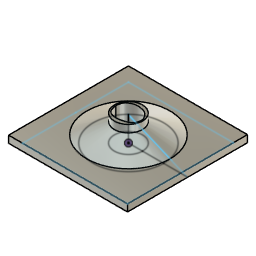
base secador v4 (Autodesk Fusion 360 design; units mm, degrees)
Autodesk Fusion 360 part; units mm, degrees
note: some values were not read from the file. Set by a fixed rule: which face or edge a step refers to.
sketch "Esboço1" plane through (0, 0, 0) normal (0, 0, 1) x (1, 0, 0)
  circle A0 centre (0, 0) radius 20
  dimension "d1" = 40
  constraint coincident A0.centre origin
  measures "d1" diameter of A0
sketch "Esboço2" plane through (0, 0, 0) normal (0, 0, 1) x (1, 0, 0)
  circle A0 centre (0, 0) radius 50
  dimension "d2" = 100
  constraint coincident A0.centre origin
  measures "d2" diameter of A0
sketch "Esboço3" plane through (0, 0, 0) normal (0, 1, 0) x (1, 0, 0)
  line L0 (0, 0) -> (82.8268, 0)
  line L1 (0, 0) -> (0, -35)
  line L2 (0, -35) -> (82.8268, 0)
  dimension "d3" = 35
  constraint coincident L0.start L1.start
  constraint horizontal L0
  constraint perpendicular L0 L1
  measures "d3" distance of L0.start L1.end
sketch "Esboço4" plane through (0, 0, 0) normal (0, 0, 1) x (1, 0, 0)
  line L0 (-75, 0) -> (-75, -75.6512)
  line L1 (-75, -75.6512) -> (74.376, -75.6512)
  line L2 (74.376, -75.6512) -> (74.376, 75.0489)
  line L3 (74.376, 75.0489) -> (-75, 75.0489)
  line L4 (-75, 75.0489) -> (-75, 0)
  constraint vertical L0
  constraint perpendicular L0 L1
  constraint perpendicular L1 L2
  constraint perpendicular L2 L3
  constraint perpendicular L1 L4
sketch "Esboço5" plane through (0, 0, 0) normal (0, 0, 1) x (1, 0, 0)
sketch "Esboço6" plane through (0, 0, 0) normal (0, 0, 1) x (1, 0, 0)
  spline S0 degree 5 poles (-18, 0) (-17.9953, 0.0513) (-17.984, 0.1676) (-17.9623, 0.4003) (-17.9267, 0.8654) (-17.8678, 1.7) (-17.7839, 2.7196) (-17.6589, 3.8334) (-17.4725, 4.9731) (-17.2029, 6.0968) (-16.8288, 7.1809) (-16.3314, 8.2159) (-15.6972, 9.2009) (-14.9196, 10.1381) (-14.0019, 11.0281) (-12.9584, 11.8645) (-11.8115, 12.6372) (-10.5887, 13.3334) (-9.3199, 13.9401) (-8.034, 14.4456) (-6.7566, 14.8417) (-5.5066, 15.1253) (-4.2932, 15.3009) (-3.115, 15.3808) (-1.9633, 15.3811) (-0.8249, 15.3201) (0.3149, 15.2144) (1.47, 15.0767) (2.6502, 14.9128) (3.8584, 14.7182) (5.0898, 14.479) (6.3344, 14.1757) (7.5785, 13.787) (8.8057, 13.293) (9.9993, 12.6789) (11.1437, 11.9389) (12.2256, 11.079) (13.236, 10.121) (14.1689, 9.0959) (15.0205, 8.0399) (15.7884, 6.9891) (16.4705, 5.9746) (17.0646, 5.0171) (17.567, 4.1233) (17.9718, 3.2782) (18.2718, 2.4505) (18.4613, 1.6037) (18.5381, 0.7059) (18.5057, -0.261) (18.3765, -1.2893) (18.1718, -2.3413) (17.917, -3.3653) (17.6378, -4.3066) (17.3549, -5.1223) (17.081, -5.7916) (16.8143, -6.3338) (16.5406, -6.8006) (16.2398, -7.2512) (15.8909, -7.7329) (15.4779, -8.2587) (14.9898, -8.8183) (14.4213, -9.3882) (13.7725, -9.9424) (13.0492, -10.4634) (12.2624, -10.9435) (11.4255, -11.3811) (10.5531, -11.7792) (9.6595, -12.1434) (8.7564, -12.4794) (7.8523, -12.7916) (6.9536, -13.0833) (6.0651, -13.3564) (5.1914, -13.6111) (4.3369, -13.846) (3.5073, -14.0577) (2.7081, -14.2417) (1.9433, -14.3944) (1.2135, -14.5139) (0.5149, -14.6018) (-0.1626, -14.6639) (-0.8314, -14.7082) (-1.5029, -14.7424) (-2.1842, -14.7713) (-2.8742, -14.7942) (-3.567, -14.8069) (-4.2556, -14.8028) (-4.9347, -14.7751) (-5.6053, -14.7179) (-6.2723, -14.6274) (-6.9419, -14.5016) (-7.6187, -14.3409) (-8.3033, -14.1483) (-8.9927, -13.9284) (-9.6826, -13.6847) (-10.3685, -13.4184) (-11.048, -13.1259) (-11.7206, -12.7985) (-12.3855, -12.4249) (-13.0395, -11.9924) (-13.676, -11.4885) (-14.2825, -10.9024) (-14.8442, -10.229) (-15.3469, -9.4714) (-15.7801, -8.6447) (-16.1399, -7.7791) (-16.4319, -6.9237) (-16.6687, -6.1307) (-16.866, -5.439) (-17.0402, -4.8597) (-17.2044, -4.3562) (-17.3662, -3.8397) (-17.5275, -3.2269) (-17.684, -2.4796) (-17.8245, -1.6706) (-17.934, -0.951) (-18.0007, -0.448) (-18.0163, -0.2501) (-18.0122, -0.1403) (-18.0047, -0.0513) (-18, 0) knots 0 0 0 0 0 0 0.00869565 0.0173913 0.02608696 0.03478261 0.04347826 0.05217391 0.06086957 0.06956522 0.07826087 0.08695652 0.09565217 0.10434783 0.11304348 0.12173913 0.13043478 0.13913043 0.14782609 0.15652174 0.16521739 0.17391304 0.1826087 0.19130435 0.2 0.20869565 0.2173913 0.22608696 0.23478261 0.24347826 0.25217391 0.26086957 0.26956522 0.27826087 0.28695652 0.29565217 0.30434783 0.31304348 0.32173913 0.33043478 0.33913043 0.34782609 0.35652174 0.36521739 0.37391304 0.3826087 0.39130435 0.4 0.40869565 0.4173913 0.42608696 0.43478261 0.44347826 0.45217391 0.46086957 0.46956522 0.47826087 0.48695652 0.49565217 0.50434783 0.51304348 0.52173913 0.53043478 0.53913043 0.54782609 0.55652174 0.56521739 0.57391304 0.5826087 0.59130435 0.6 0.60869565 0.6173913 0.62608696 0.63478261 0.64347826 0.65217391 0.66086957 0.66956522 0.67826087 0.68695652 0.69565217 0.70434783 0.71304348 0.72173913 0.73043478 0.73913043 0.74782609 0.75652174 0.76521739 0.77391304 0.7826087 0.79130435 0.8 0.80869565 0.8173913 0.82608696 0.83478261 0.84347826 0.85217391 0.86086957 0.86956522 0.87826087 0.88695652 0.89565217 0.90434783 0.91304348 0.92173913 0.93043478 0.93913043 0.94782609 0.95652174 0.96521739 0.97391304 0.9826087 0.99130435 1 1 1 1 1 1
  point P0 (-17.7489, 2.9823)
  point P1 (-15, 10)
  point P2 (-6, 15)
  point P3 (2, 15)
  point P4 (11, 12)
  point P5 (17.2384, 4.6936)
  point P6 (18.5, 0)
  point P7 (17.2407, -5.3862)
  point P8 (16.2247, -7.2631)
  point P9 (14.2609, -9.5114)
  point P10 (10, -12)
  point P11 (5.072, -13.6412)
  point P12 (1.252, -14.5016)
  point P13 (-1.5356, -14.7425)
  point P14 (-4.3539, -14.7942)
  point P15 (-7.0748, -14.4644)
  point P16 (-10.0019, -13.5574)
  point P17 (-13, -12)
  point P18 (-15.7735, -8.6103)
  point P19 (-17, -5)
  point P20 (-17.5874, -2.9212)
  point P21 (-18, -0.4064)
revolve "Revolucionar1" add sketch "Esboço3" angle 360 about axis through (0, 0, 0) along (0, 0, 1)
extrude "Extrusão2" cut sketch "Esboço1" along normal blind 37
extrude "Extrusão3" add sketch "Esboço1" along normal blind 37
extrude "Extrusão4" cut sketch "Esboço6" along normal blind 37
extrude "Extrusão5" add sketch "Esboço4" along normal blind 10
extrude "Extrusão6" add 1 faces at (1.1659, 16.6843, 37) along direction (0, 0, 1) blind 10
extrude "Extrusão7" cut 1 faces at (1.1659, 16.6843, 47) along direction (0, 0, -1) blind 10
extrude "Extrusão8" add 1 faces at (74.376, -62.5836, 3.3333) along direction (1, 0, 0) blind 10
extrude "Extrusão9" add 2 faces at (77.7094, 75.0489, 3.3333) (-61.6807, 75.0489, 3.3333) along direction (0, 1, 0) blind 10
extrude "Extrusão10" add 2 faces at (77.7094, -75.6512, 3.3333) (-61.2407, -75.6512, 3.3333) along direction (0, -1, 0) blind 10
extrude "Extrusão11" add 4 faces at (-75, -78.9845, 3.3333) (-75, -62.1497, 3.3333) (-75, 61.7481, 3.3333) (-75, 78.3822, 3.3333) along direction (-1, 0, 0) blind 10
extrude "Extrusão12" add 10 faces at (-78.3333, -78.9845, 10) (-78.3333, -25.2171, 10) (-78.3333, 50.0326, 10) (-81.6667, 78.3822, 10) (-25.208, -78.9845, 10) (77.7094, -78.9845, 10) (-67.7677, -33.7736, 10) (24.584, 78.3822, 10) (81.0427, -25.4178, 10) (77.7094, 78.3822, 10) along direction (0, 0, -1) blind 10
